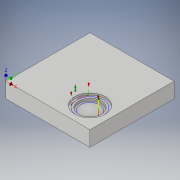
# Autodesk Inventor part: Saber plaque
Saved by Autodesk Inventor 2017 SP1 (Build 210196100, 196)
## iProperties
Created: 2017-11-06
Part Number: Saber plaque
Material: Generic
Document SubType Name: Modeling
Designer: rmainhar
Density: 1 g/cm^3
Appearance: Default
Author: rmainhar
Autodesk Inventor part; units mm, degrees
ref_plane "YZ Plane" through (0, 0, 0) normal (1, 0, 0) x (0, 1, 0)
ref_plane "XZ Plane" through (0, 0, 0) normal (0, 1, 0) x (-1, 0, 0)
ref_plane "XY Plane" through (0, 0, 0) normal (0, 0, 1) x (1, 0, 0)
sketch "Sketch1" plane through (0, 0, 0) normal (0, 1, 0) x (-1, 0, 0)
  line L0 (0, 0) -> (-139.7, 0)
  line L1 (-139.7, 0) -> (-139.7, -139.7)
  line L2 (-139.7, -139.7) -> (0, -139.7)
  line L3 (0, -139.7) -> (0, 0)
  dimension "d0" = 139.7
  dimension "d1" = 139.7
  constraints: 8 end point, 2 parallel, 1 horizontal, 1 perpendicular
  measures "d0" distance of L2.end L1.end
  measures "d1" distance of L1.end L0.end
extrude "Extrusion1" add sketch "Sketch1" along normal blind 25.4
sketch "Sketch2" plane through (0, 25.4, 0) normal (0, 1, 0) x (1, 0, 0)
  circle A0 centre (104.775, 34.925) radius 25.4
  line L0 (0, 0) -> (139.7, 0) projected
  line L1 (139.7, 0) -> (139.7, 139.7) projected
  line L2 (139.7, 139.7) -> (0, 139.7) projected
  line L3 (0, 139.7) -> (0, 0) projected
  dimension "d4" = 50.8
  dimension "d5" = 34.925
  dimension "d6" = 34.925
  constraints: 1 centre point
  measures "d4" diameter of A0
  measures "d5" horizontal distance of A0.centre L0.end
  measures "d6" distance from line of L0 A0.centre
extrude "Extrusion2" cut sketch "Sketch2" against normal blind 3.175 contours A0
sketch "Sketch3" plane through (104.775, 22.225, -34.925) normal (0, 1, 0) x (1, 0, 0)
  circle A0 centre (0, 0) radius 19.05
  point P0 (-104.775, -34.925)
  dimension "d9" = 38.1
  constraints: 1 centre point
  measures "d9" diameter of A0
extrude "Extrusion3" cut sketch "Sketch3" against normal blind 3.937
equation "\"d5\" = d6"
body "Solid1"
